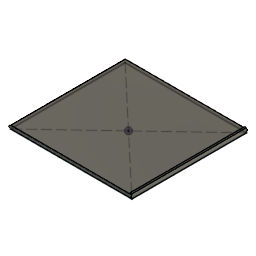
lid (Autodesk Fusion 360 design; units mm, degrees)
part number: 2026-05-05-14-56-08-613
part number: 2026-05-05-14-58-18-164
Autodesk Fusion 360 part; units mm, degrees
sketch "Sketch1" plane through (0, 0, 0) normal (0, 0, 1) x (1, 0, 0) in component "lid"
  line L0 (-54, 51) -> (54, 51)
  line L1 (54, 51) -> (54, -51)
  line L2 (54, -51) -> (-54, -51)
  line L3 (-54, -51) -> (-54, 51)
  line L4 (-54, 51) -> (54, -51) construction
  line L5 (54, 51) -> (-54, -51) construction
  dimension "d1" = 108
  dimension "d2" = 102
  constraint horizontal L0
  constraint perpendicular L0 L1
  constraint parallel L0 L2
  constraint parallel L1 L3
  constraint coincident L4 origin
  constraint coincident L5 origin
  measures "d1" distance of L1.end L2.end
  measures "d2" distance of L0.end L1.end
extrude "Extrude1" add sketch "Sketch1" along normal blind 3 in component "lid"
sketch "Sketch2" plane through (0, 0, 3) normal (0, 0, 1) x (-1, 0, 0) in component "lid"
  line L0 (54, 51) -> (-54, 51)
  line L1 (-54, 51) -> (-54, -51)
  line L2 (-54, -51) -> (54, -51)
  line L3 (54, -51) -> (54, 51)
  line L4 (-54, 51) -> (-52, 51)
  line L5 (-52, 51) -> (-52, -51)
  line L6 (-52, -51) -> (-54, -51)
  line L7 (-54, -51) -> (-54, 51)
  dimension "d5" = 2
  dimension "d6" = 102
  constraint horizontal L4
  constraint vertical L5
  constraint horizontal L6
  constraint vertical L7
  constraint coincident L0.end L1.start
  measures "d5" distance of L0.end L4.end
  measures "d6" distance of L0.end L1.end
extrude "Extrude2" add sketch "Sketch2" along normal blind 1 contours L0 L1 L2 L4 L5 L6 L7 in component "lid"
sketch "Sketch3" plane through (54, 0, 0) normal (1, 0, 0) x (0, 1, 0) in component "lid"
  line L0 (-51, 0) -> (51, 0)
  line L1 (51, 0) -> (51, 4)
  line L2 (51, 4) -> (-51, 4)
  line L3 (-51, 4) -> (-51, 0)
  line L4 (-51, 0) -> (-51, 4) construction
  line L5 (-51, 0, -108) -> (-51, 3, -108)
  line L6 (-51, 2, 0) -> (-51, 2, -108)
  line L7 (-51, 3, -108) -> (-51, 3, -2)
  line L8 (51, 0, -108) -> (51, 3, -108)
  line L9 (-51, 2, -108) -> (51, 2, -108)
  line L10 (51, 2, -108) -> (51, 2, 0)
  line L11 (51, 3, -108) -> (-51, 3, -108)
  line L12 (51, 3, -2) -> (51, 3, -108)
  arc A0 (-51, 2.9) -> (-51, 1.1) centre (-51, 2) ccw
  dimension "d18" = 1.8
  dimension "d19" = 0.9
  constraint coincident L0.start L3.end
  constraint coincident L2.end L3.start
  constraint coincident L4 A0.start
  constraint coincident L4 A0.end
  measures "d18" distance of A0.start A0.end
  measures "d19" radius of A0
sweep "Sweep1" add profiles "Sketch3" path "Sketch3" along L6 L9 L10 section 1 contours L3 A0 in component "lid"
fillet "Fillet1" radius 0.2 2 edges at (-54.9, 51.9, 2) (-54.9, -51.9, 2) in component "lid"
fillet "Fillet1" radius 0.4 3 edges at (-54, -51, 0.55) (-54, 51, 0.55) (-54, 0, 3) in component "lid"
fillet "Fillet1" radius 0.4 3 edges at (52, 51, 3.5) (52, 0, 4) (52, -51, 3.5) in component "lid"
component "lid" placed x (1, 0, 0) y (0, 1, 0) z (0, 0, 1) at (0, 0, 0)
